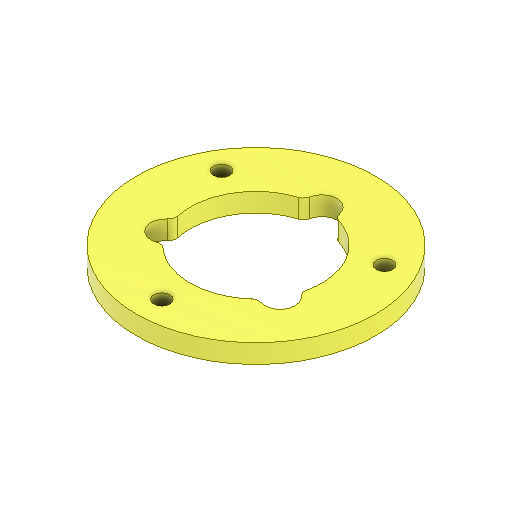
# Autodesk Inventor part: B_probe_bearing
Saved by Autodesk Inventor 2026.2 (Build 302298000, 298)
## iProperties
Created: 2026-06-04
Part Number: B_probe_bearing
Material: PAEK 樹脂
Document SubType Name: Modeling
Designer: zetsu
Density: 1.32 g/cm^3
Appearance: 滑らか - 黄
Author: zetsu
Autodesk Inventor part; units mm, degrees
ref_plane "YZ Plane" through (0, 0, 0) normal (1, 0, 0) x (0, 1, 0)
ref_plane "XZ Plane" through (0, 0, 0) normal (0, 1, 0) x (-1, 0, 0)
ref_plane "XY Plane" through (0, 0, 0) normal (0, 0, 1) x (1, 0, 0)
sketch "スケッチ1" plane through (0, 0, 0) normal (0, 1, 0) x (-1, 0, 0)
  circle A0 centre (0, 0) radius 31.75
  dimension "d0" = 63.5
  constraints: 1 centre point, 1 coincident
  measures "d0" diameter of A0
extrude "押し出し1" add sketch "スケッチ1" along normal blind 5
sketch "スケッチ4" plane through (0, 5, 0) normal (0, 1, 0) x (1, 0, 0)
  circle A0 centre (0, 0) radius 17.5
  dimension "d9" = 35
  constraints: 1 centre point, 1 coincident
  measures "d9" diameter of A0
extrude "押し出し4" cut sketch "スケッチ4" against normal through all
sketch "スケッチ5" plane through (0, 5, 0) normal (0, 1, 0) x (1, 0, 0)
  circle A0 centre (0, 0) radius 17.5 projected
  circle A1 centre (0, 17.5) radius 4
  circle A2 centre (-15.1554, -8.75) radius 4
  circle A3 centre (15.1554, -8.75) radius 4
  point P0 (3.9738, 17.0429)
  point P1 (-3.9738, 17.0429)
  point P2 (-12.7727, -11.9628)
  point P3 (-16.7464, -5.08)
  point P4 (12.7727, -11.9628)
  point P5 (16.7464, -5.08)
  dimension "d12" = 8
  dimension "d30" = 360
  constraints: 3 centre point, 9 other
  measures "d12" diameter of A1
extrude "押し出し5" cut sketch "スケッチ5" against normal through all contours A0 A1 | A3 A0 | A0 A2 picked at (-0.0763, 18.7972) picked at (16.3019, -9.3615) picked at (-16.2807, -9.3997)
sketch "スケッチ6" plane through (0, 5, 0) normal (0, 1, 0) x (1, 0, 0)
  circle A0 centre (0, 0) radius 25 construction
  circle A1 centre (21.6506, 12.5) radius 2.15
  line L0 (0, 0) -> (21.6506, 12.5) construction
  line L1 (0, 0) -> (35.9214, 0) construction
  circle A2 centre (-21.6506, 12.5) radius 2.15
  circle A3 centre (0, -25) radius 2.15
  dimension "d19" = 50
  dimension "d20" = 4.3
  dimension "d21" = 30
  dimension "d24" = 360
  constraints: 4 end point, 3 centre point, 1 coincident, 1 horizontal, 10 other
  measures "d20" diameter of A1
  measures "d21" angle of L1 L0
extrude "押し出し6" cut sketch "スケッチ6" against normal through all
fillet "フィレット1" radius 2 6 edges at (-3.9738, 2.5, -17.0429) (3.9738, 2.5, -17.0429) (16.7464, 2.5, 5.08) (12.7727, 2.5, 11.9628) (-12.7727, 2.5, 11.9628) (-16.7464, 2.5, 5.08)
